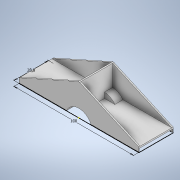
# Autodesk Inventor part: kolyska_v2
Saved by Autodesk Inventor 2020.3 (Build 243373000, 373)
## iProperties
Created: 2020-12-18
Part Number: kolyska_v2
Material: Ogólny
Document SubType Name: Modeling
Designer: sitar
Density: 1 g/cm^3
Appearance: Domyślna
Author: sitar
Autodesk Inventor part; units mm, degrees
ref_plane "YZ Plane" through (0, 0, 0) normal (1, 0, 0) x (0, 1, 0)
ref_plane "XZ Plane" through (0, 0, 0) normal (0, 1, 0) x (-1, 0, 0)
ref_plane "XY Plane" through (0, 0, 0) normal (0, 0, 1) x (1, 0, 0)
sketch "Szkic1" plane through (0, 0, 0) normal (0, 1, 0) x (-1, 0, 0)
  point P0 (0, 0)
sketch "Szkic2" plane through (0, 0, 0) normal (0, 1, 0) x (-1, 0, 0)
  line L0 (50, -14.4) -> (-50, -14.4)
  line L1 (-50, -14.4) -> (-50, 14.4)
  line L2 (-50, 14.4) -> (50, 14.4)
  line L3 (50, 14.4) -> (50, -14.4)
  line L4 (50, -14.4) -> (-50, 14.4) construction
  line L5 (-50, -14.4) -> (50, 14.4) construction
  point P0 (0, 0)
  dimension "d0" = 100
  dimension "d1" = 28.8
  constraints: 12 end point, 2 midpoint, 2 parallel, 1 horizontal, 1 perpendicular
  measures "d0" distance of L1.end L2.end
  measures "d1" distance of L0.end L1.end
extrude "Wyciągnięcie proste1" add sketch "Szkic2" along normal blind 4
sketch "Szkic3" plane through (0, 4, 0) normal (0, 1, 0) x (1, 0, 0)
  line L0 (-0.6, 14.4) -> (0.6, 14.4)
  line L1 (0.6, 14.4) -> (0.6, -14.4)
  line L2 (0.6, -14.4) -> (-0.6, -14.4)
  line L3 (-0.6, -14.4) -> (-0.6, 14.4)
  line L4 (-0.6, 14.4) -> (0.6, -14.4) construction
  line L5 (0.6, 14.4) -> (-0.6, -14.4) construction
  point P0 (0, 0)
  dimension "d4" = 1.2
  dimension "d5" = 28.8
  constraints: 12 end point, 2 midpoint, 2 parallel, 1 horizontal, 1 perpendicular
  measures "d4" distance of L1.end L2.end
  measures "d5" distance of L0.end L1.end
extrude "Wyciągnięcie proste2" add sketch "Szkic3" along normal blind 22
sketch "Szkic4" plane through (-50, 0, 14.4) normal (0, 0, 1) x (1, 0, 0)
  line L0 (0, 0) -> (0, 4) projected
  line L1 (50.6, 26) -> (49.4, 26) projected
  line L2 (0, 4) -> (49.4, 26)
  line L3 (0, 4) -> (49.4, 4) projected
  line L4 (49.4, 26) -> (49.4, 4)
  line L5 (49.4, 4) -> (0, 4)
  point P0 (50, 0)
  constraints: 6 end point, 2 perpendicular
extrude "Wyciągnięcie proste3" add sketch "Szkic4" against normal blind 1.2
mirror "Odbij1" about plane through (0, 0, 0) normal (1, 0, 0) of "Wyciągnięcie proste3"
mirror "Odbij2" about plane through (0, 0, 0) normal (0, 0, 1) of "Wyciągnięcie proste3", "Odbij1"
sketch "Szkic5" plane through (-50, 0, 14.4) normal (0, 0, 1) x (1, 0, 0)
  point P0 (50, 0)
sketch "Szkic6" plane through (-50, 0, 14.4) normal (0, 0, 1) x (1, 0, 0)
  line L0 (50, 0) -> (50, -3)
  circle A0 centre (50, -3) radius 11.6
  dimension "d10" = 3
  dimension "d11" = 23.2
  constraints: 2 end point, 1 centre point, 1 coincident, 1 vertical
  measures "d10" distance of L0.start L0.end
  measures "d11" diameter of A0
extrude "Wyciągnięcie proste4" add sketch "Szkic6" against normal blind 8
sketch "Szkic7" plane through (-50, 0, 14.4) normal (0, 0, 1) x (1, 0, 0)
  line L0 (50, 0) -> (50, -4)
  circle A0 centre (50, -4) radius 11
  dimension "d14" = 4
  dimension "d15" = 22
  constraints: 2 end point, 1 centre point, 1 coincident, 1 vertical
  measures "d14" distance of L0.start L0.end
  measures "d15" diameter of A0
extrude "Wyciągnięcie proste5" cut sketch "Szkic7" against normal blind 6.8
mirror "Odbij3" about plane through (0, 0, 0) normal (0, 0, 1) of "Wyciągnięcie proste4", "Wyciągnięcie proste5"
sketch "Szkic8" plane through (0, 0, 0) normal (0, -1, 0) x (1, 0, 0)
  line L0 (50, -14.4) -> (-50, -14.4)
  line L1 (-50, -14.4) -> (-50, 14.4)
  line L2 (-50, 14.4) -> (50, 14.4)
  line L3 (50, 14.4) -> (50, -14.4)
  line L4 (50, -14.4) -> (-50, 14.4) construction
  line L5 (-50, -14.4) -> (50, 14.4) construction
  point P0 (0, 0)
  dimension "d18" = 100
  dimension "d19" = 28.8
  constraints: 12 end point, 2 midpoint, 2 parallel, 1 horizontal, 1 perpendicular
  measures "d18" distance of L1.end L2.end
  measures "d19" distance of L0.end L1.end
extrude "Wyciągnięcie proste6" cut sketch "Szkic8" along normal through all
sketch "Szkic9" plane through (0, 0, 0) normal (0, -1, 0) x (1, 0, 0)
  line L0 (50, 14.4) -> (50, -14.4) projected
  line L1 (50, 0) -> (43, 0)
  line L2 (36, -14) -> (50, -14)
  line L3 (50, -14) -> (50, 14)
  line L4 (50, 14) -> (36, 14)
  line L5 (36, 14) -> (36, -14)
  line L6 (36, -14) -> (50, 14) construction
  line L7 (50, -14) -> (36, 14) construction
  point P0 (0, 0)
  point P1 (50, -14)
  point P2 (50, 14)
  dimension "d22" = 7
  dimension "d23" = 14
  dimension "d24" = 28
  constraints: 14 end point, 3 midpoint, 2 horizontal, 2 parallel, 1 perpendicular
  measures "d22" distance of L1.start L1.end
  measures "d23" distance of L4.end L3.end
  measures "d24" distance of L3.end L2.end
extrude "Wyciągnięcie proste7" cut sketch "Szkic9" against normal blind 2.8
mirror "Odbij4" about plane through (0, 0, 0) normal (1, 0, 0) of "Wyciągnięcie proste7"
sketch "Szkic10" plane through (0, 0, 0) normal (0, -1, 0) x (1, 0, 0)
  line L0 (50, -14.4) -> (-50, -14.4)
  line L1 (-50, -14.4) -> (-50, 14.4)
  line L2 (-50, 14.4) -> (50, 14.4)
  line L3 (50, 14.4) -> (50, -14.4)
  line L4 (50, -14.4) -> (-50, 14.4) construction
  line L5 (-50, -14.4) -> (50, 14.4) construction
  point P0 (0, 0)
  dimension "d27" = 100
  dimension "d28" = 28.8
  constraints: 12 end point, 2 midpoint, 2 parallel, 1 horizontal, 1 perpendicular
  measures "d27" distance of L1.end L2.end
  measures "d28" distance of L0.end L1.end
sketch "Szkic11" plane through (0, 0, 0) normal (0, -1, 0) x (1, 0, 0)
  line L0 (-50, 14.4) -> (50, 14.4)
  line L1 (50, 14.4) -> (50, -14.4)
  line L2 (50, -14.4) -> (-50, -14.4)
  line L3 (-50, -14.4) -> (-50, 14.4)
  line L4 (-50, 14.4) -> (50, -14.4) construction
  line L5 (50, 14.4) -> (-50, -14.4) construction
  point P0 (0, 0)
  dimension "d29" = 100
  dimension "d30" = 28.8
  constraints: 12 end point, 2 midpoint, 2 parallel, 1 horizontal, 1 perpendicular
  measures "d29" distance of L1.end L2.end
  measures "d30" distance of L0.end L1.end
extrude "Wyciągnięcie proste8" cut sketch "Szkic11" against normal blind 0.4
